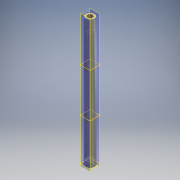
# Autodesk Inventor part: 殷钢管
Saved by Autodesk Inventor 2016 (Build 200138000, 138)
## iProperties
Created: 2017-07-28
Part Number: 殷钢管
Material: 钢，合金
Document SubType Name: Modeling
Designer: Administrator
Density: 7.73 g/cm^3
Appearance: 半抛光
Author: Administrator
Autodesk Inventor part; units mm, degrees
ref_plane "YZ Plane" through (0, 0, 0) normal (1, 0, 0) x (0, 1, 0)
sketch "草图1" plane through (0, 0, 0) normal (0, 0, 1) x (1, 0, 0)
  circle A0 centre (0, 0) radius 12.5
  dimension "d0" = 25
  constraints: 1 centre point, 1 coincident
  measures "d0" diameter of A0
extrude "拉伸1" add sketch "草图1" along normal mid plane 350
ref_plane "工作平面1" through (0, 0, 175) normal (0, 0, 1) x (1, 0, 0)
ref_plane "工作平面3" through (0, 0, -165) normal (0, 0, 1) x (1, 0, 0)
sketch "草图2" plane through (0, 0, 175) normal (0, 0, 1) x (1, 0, 0)
  circle A0 centre (0, 0) radius 6.5
  dimension "d64" = 13
  constraints: 1 centre point, 1 coincident
  measures "d64" diameter of A0
sketch "草图3" plane through (0, 0, -165) normal (0, 0, 1) x (1, 0, 0)
  circle A0 centre (0, 0) radius 4.5
  circle A1 centre (0, 0) radius 6.5
  dimension "d15" = 9
  dimension "d16" = 13
  constraints: 2 centre point
  measures "d15" diameter of A0
  measures "d16" diameter of A1
extrude "拉伸2" cut sketch "草图3" along normal blind 350 contours A0
ref_plane "工作平面4" through (0, 12.5, 0) normal (0, 1, 0) x (-1, 0, 0)
sketch "草图8" plane through (0, 0, 175) normal (0, 0, 1) x (1, 0, 0)
  circle A0 centre (0, 0) radius 6.5 projected
  circle A1 centre (0, 6.5) radius 1.5
  dimension "d37" = 3
  constraints: 1 centre point, 1 vertical alignment, 1 other
  measures "d37" diameter of A1
ref_plane "工作平面5" through (0, -12.5, 0) normal (0, 1, 0) x (-1, 0, 0)
sketch "草图9" plane through (0, -12.5, 0) normal (0, 1, 0) x (-1, 0, 0)
  point P0 (0, 0)
  point P1 (0, 0)
  point P2 (0, 60)
  point P3 (0, -60)
  dimension "d41" = 60
  dimension "d42" = 60
  constraints: 1 coincident
  measures "d41" distance of point (0, 60) point (0, 0)
  measures "d42" distance of point (0, 0) point (0, -60)
hole "孔3" at (0, -12.5, 60) at (0, -12.5, -60) direction (0, 1, 0) diameter 2.459 depth 8.8 tip angle 118 thread size "M3x0.5" designation "M3" class "6H" standard "GB Metric profile"
ref_plane "工作平面6" through (0, 0, 60) normal (0, 0, 1) x (1, 0, 0)
sketch "草图11" plane through (0, 0, 60) normal (0, 0, 1) x (1, 0, 0)
  line L0 (0, 0) -> (0, -12.3)
  line L1 (2.2271, -12.3) -> (-2.2271, -12.3)
  arc A0 (2.2271, -12.3) -> (0, 12.5) centre (0, 0) ccw
  arc A1 (0, 12.5) -> (-2.2271, -12.3) centre (0, 0) ccw
  circle A2 centre (0, 0) radius 12.5
  constraints: 4 end point, 4 point on circle, 3 centre point, 2 coincident, 1 concentric, 1 midpoint, 1 perpendicular, 1 point on line, 1 vertical
extrude "拉伸6" cut sketch "草图11" along normal mid plane 20 contours A2 L1
ref_plane "工作平面7" through (0, 0, -60) normal (0, 0, 1) x (1, 0, 0)
sketch "草图12" plane through (0, 0, -60) normal (0, 0, 1) x (1, 0, 0)
  line L0 (0, 0) -> (0, -12.3)
  line L1 (2.2271, -12.3) -> (-2.2271, -12.3)
  arc A0 (2.2271, -12.3) -> (0, 12.5) centre (0, 0) ccw
  arc A1 (0, 12.5) -> (-2.2271, -12.3) centre (0, 0) ccw
  circle A2 centre (0, 0) radius 12.5
  constraints: 4 end point, 4 point on circle, 3 centre point, 2 coincident, 1 concentric, 1 midpoint, 1 perpendicular, 1 point on line, 1 vertical
extrude "拉伸7" cut sketch "草图12" along normal mid plane 20 contours A2 L1
ref_plane "工作平面8" through (0, 0, -175) normal (0, 0, 1) x (1, 0, 0)
sketch "草图13" plane through (0, 0, -175) normal (0, 0, 1) x (1, 0, 0)
  circle A0 centre (0, 0) radius 6.5
  dimension "d59" = 13
  constraints: 1 centre point, 1 coincident
  measures "d59" diameter of A0
extrude "拉伸8" cut sketch "草图13" along normal blind 15
extrude "拉伸9" cut sketch "草图2" against normal blind 36
thread "螺纹3" size "M14x0.5" class "6H" standard "GB Metric profile" full length
thread "螺纹5" size "M14x0.5" class "6H" standard "ANSI Metric M Profile" full length
extrude "拉伸10" cut sketch "草图8" against normal blind 36 contours A1 A0 | A0 A1 picked at (0, 5.9871) picked at (-0.0289, 6.9863)
